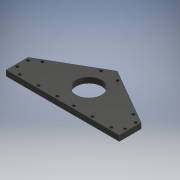
# Autodesk Inventor part: HB04
Saved by Autodesk Inventor 2017 (Build 210142000, 142)
## iProperties
Created: 2019-05-20
Part Number: HB04
Material: Polyethylene, High Density
Document SubType Name: Modeling
Designer: Dell
Density: 0.952 g/cm^3
Appearance: Smooth - Black
Mass: 1258.66 g
Surface Area: 2467.82 cm^2
Volume: 1322.13 cm^3
Author: Dell
Autodesk Inventor part; units mm, degrees
ref_plane "YZ Plane" through (0, 0, 0) normal (1, 0, 0) x (0, 1, 0)
ref_plane "XZ Plane" through (0, 0, 0) normal (0, 1, 0) x (-1, 0, 0)
ref_plane "XY Plane" through (0, 0, 0) normal (0, 0, 1) x (1, 0, 0)
sketch "Sketch1" plane through (0, 0, 0) normal (0, 0, 1) x (1, 0, 0)
  line L0 (262.89, 253.3796) -> (525.78, 101.6)
  line L1 (525.78, 101.6) -> (525.78, -201.9592) construction
  line L2 (525.78, -201.9592) -> (262.89, -353.7388) construction
  line L3 (262.89, -353.7388) -> (0, -201.9592) construction
  line L4 (0, -201.9592) -> (0, 101.6) construction
  line L5 (0, 101.6) -> (262.89, 253.3796)
  line L6 (0, 101.6) -> (0, 0)
  line L7 (0, 0) -> (525.78, 0)
  line L8 (525.78, 0) -> (525.78, 101.6)
  point P0 (262.89, -50.1796)
  dimension "d0" = 525.78
  dimension "d1" = 101.6
  constraints: 18 end point, 2 collinear, 2 point on line, 1 perpendicular, 1 vertical, 13 other
  measures "d0" distance between parallel lines of L4 L1
  measures "d1" distance of L6.end L4.end
extrude "Extrusion1" add sketch "Sketch1" along normal blind 25.4
sketch "Sketch2" plane through (0, 0, 25.4) normal (0, 0, 1) x (1, 0, 0)
  circle A0 centre (262.89, 121.3796) radius 60
  line L0 (0, 0) -> (525.78, 0) projected
  point P0 (262.89, 0)
  dimension "d4" = 121.3796
  dimension "d5" = 120
  constraints: 1 centre point, 1 midpoint, 1 vertical alignment
  measures "d4" distance from line of L0 A0.centre
  measures "d5" diameter of A0
extrude "Extrusion2" cut sketch "Sketch2" against normal through all
sketch "Sketch3" plane through (0, 0, 25.4) normal (0, 0, 1) x (1, 0, 0)
  circle A0 centre (262.89, 121.3796) radius 60 construction
  line L0 (0, 101.6) -> (0, 0) construction
  line L1 (0, 0) -> (525.78, 0) construction
  line L2 (525.78, 0) -> (525.78, 101.6) construction
  line L3 (525.78, 101.6) -> (262.89, 253.3796) construction
  line L4 (262.89, 253.3796) -> (0, 101.6) construction
  line L5 (12.7, 94.2677) -> (12.7, 12.7) construction
  line L6 (12.7, 12.7) -> (513.08, 12.7) construction
  line L7 (513.08, 12.7) -> (513.08, 94.2677) construction
  line L8 (513.08, 94.2677) -> (262.89, 238.7149) construction
  line L9 (262.89, 238.7149) -> (12.7, 94.2677) construction
  circle A1 centre (12.7, 88.5) radius 2
  circle A2 centre (12.7, 38.5) radius 2
  line L10 (12.7, 88.5) -> (12.7, 38.5) construction
  circle A3 centre (51.1925, 116.4913) radius 2
  circle A4 centre (224.3975, 216.4913) radius 2
  circle A5 centre (137.795, 166.4913) radius 2
  circle A6 centre (51.1925, 12.7) radius 2
  circle A7 centre (137.795, 12.7) radius 2
  circle A8 centre (224.3975, 12.7) radius 2
  circle A9 centre (262.89, 12.7) radius 2
  line L11 (51.1925, 116.4913) -> (224.3975, 216.4913) construction
  line L12 (262.89, 238.7149) -> (262.89, 253.3796)
  line L13 (525.78, 101.6) -> (525.78, 0) construction
  line L14 (513.08, 94.2677) -> (513.08, 12.7) construction
  circle A10 centre (513.08, 88.5) radius 2
  circle A11 centre (513.08, 38.5) radius 2
  line L15 (513.08, 88.5) -> (513.08, 38.5) construction
  circle A12 centre (474.5875, 116.4913) radius 2
  circle A13 centre (301.3825, 216.4913) radius 2
  circle A14 centre (387.985, 166.4913) radius 2
  circle A15 centre (474.5875, 12.7) radius 2
  circle A16 centre (387.985, 12.7) radius 2
  circle A17 centre (301.3825, 12.7) radius 2
  circle A18 centre (262.89, 12.7) radius 2
  line L16 (474.5875, 116.4913) -> (301.3825, 216.4913) construction
  line L17 (30.0651, 0) -> (30.0651, 25.4)
  line L18 (30.0651, 25.4) -> (30.0651, 101.6)
  point P0 (525.78, 0)
  point P1 (30.0651, 63.5)
  point P2 (12.7, 63.5)
  dimension "d8" = 12.7
  dimension "d9" = 4
  dimension "d10" = 4
  dimension "d11" = 50
  dimension "d12" = 4
  dimension "d13" = 4
  dimension "d14" = 4
  dimension "d15" = 4
  dimension "d16" = 4
  dimension "d17" = 4
  dimension "d18" = 4
  dimension "d19" = 200
  dimension "d38" = 25.4
  constraints: 28 end point, 18 centre point, 10 point on line, 9 symmetric about line, 5 midpoint, 3 vertical alignment, 2 collinear, 2 horizontal alignment, 2 vertical, 1 perpendicular, 13 other
  measures "d8" distance between parallel lines of L4 L9
  measures "d9" diameter of A1
  measures "d10" diameter of A2
  measures "d11" distance of L10.end L10.start
  measures "d12" diameter of A3
  measures "d13" diameter of A4
  measures "d14" diameter of A5
  measures "d15" diameter of A6
  measures "d16" diameter of A7
  measures "d17" diameter of A8
  measures "d18" diameter of A9
  measures "d19" distance of L11.start L11.end
  measures "d38" distance of L17.start L17.end
extrude "Extrusion3" cut sketch "Sketch3" against normal through all contours A1 | A2 | A3 | A4 | A7 | A8 | A10 | A11 | A12 | A13 | A16 | A17
sketch "Sketch5" plane through (0, 0, 0) normal (0, 0, -1) x (-1, 0, 0)
  circle A0 centre (-513.08, 88.5) radius 2 projected
  circle A1 centre (-387.985, 12.7) radius 2 projected
  circle A2 centre (-224.3975, 216.4913) radius 2 projected
  circle A3 centre (-12.7, 38.5) radius 2 projected
  circle A4 centre (-12.7, 88.5) radius 2 projected
  circle A5 centre (-51.1925, 116.4913) radius 2 projected
  circle A6 centre (-137.795, 12.7) radius 2 projected
  circle A7 centre (-301.3825, 216.4913) radius 2 projected
  circle A8 centre (-474.5875, 116.4913) radius 2 projected
  circle A9 centre (-513.08, 38.5) radius 2 projected
  circle A10 centre (-262.89, 121.3796) radius 60 projected
  line L0 (0, 0) -> (0, 101.6) projected
  line L1 (0, 101.6) -> (-262.89, 253.3796) projected
  line L2 (-262.89, 253.3796) -> (-525.78, 101.6) projected
  line L3 (-525.78, 101.6) -> (-525.78, 0) projected
  line L4 (-525.78, 0) -> (0, 0) projected
  line L5 (-25.4, 25.4) -> (-25.4, 86.9353)
  line L6 (-25.4, 86.9353) -> (-262.89, 224.0502)
  line L7 (-262.89, 224.0502) -> (-500.38, 86.9353)
  line L8 (-500.38, 86.9353) -> (-500.38, 25.4)
  line L9 (-500.38, 25.4) -> (-25.4, 25.4)
  circle A11 centre (-262.89, 121.3796) radius 85.4
  dimension "d26" = 25.4
  dimension "d27" = 25.4
  constraints: 10 end point, 1 centre point, 4 other
  measures "d26" distance between parallel lines of L4 L9
  measures "d27" radial gap between concentric circles of A10 A11
extrude "Extrusion5" cut sketch "Sketch5" against normal blind 19.05 contours L9 L8 L7 L6 L5
sketch "Sketch6" plane through (0, 0, 25.4) normal (0, 0, 1) x (1, 0, 0)
  circle A0 centre (513.08, 38.5) radius 2 construction
  circle A1 centre (513.08, 88.5) radius 2 construction
  circle A2 centre (387.985, 12.7) radius 2 construction
  circle A3 centre (224.3975, 216.4913) radius 2 construction
  circle A4 centre (12.7, 38.5) radius 2 construction
  circle A5 centre (12.7, 88.5) radius 2 construction
  circle A6 centre (51.1925, 116.4913) radius 2 construction
  circle A7 centre (137.795, 12.7) radius 2 construction
  circle A8 centre (301.3825, 216.4913) radius 2 construction
  circle A9 centre (474.5875, 116.4913) radius 2 construction
  circle A10 centre (513.08, 38.5) radius 2 construction
  circle A11 centre (262.89, 121.3796) radius 60 construction
  line L0 (0, 101.6) -> (0, 0) construction
  line L1 (0, 0) -> (525.78, 0) construction
  line L2 (525.78, 0) -> (525.78, 101.6) construction
  line L3 (525.78, 101.6) -> (262.89, 253.3796) construction
  line L4 (262.89, 253.3796) -> (0, 101.6) construction
  circle A12 centre (513.08, 38.5) radius 2 projected
  circle A13 centre (513.08, 38.5) radius 6.5
  circle A14 centre (513.08, 88.5) radius 2 projected
  circle A15 centre (513.08, 88.5) radius 6.5
  circle A16 centre (474.5875, 116.4913) radius 2 projected
  circle A17 centre (474.5875, 116.4913) radius 6.5
  circle A18 centre (301.3825, 216.4913) radius 2 projected
  circle A19 centre (301.3825, 216.4913) radius 6.5
  circle A20 centre (387.985, 12.7) radius 2 projected
  circle A21 centre (387.985, 12.7) radius 6.5
  line L5 (262.89, 253.3796) -> (262.89, 364.4597)
  circle A22 centre (12.7, 88.5) radius 2 construction
  circle A23 centre (12.7, 38.5) radius 6.5
  circle A24 centre (12.7, 88.5) radius 6.5
  circle A25 centre (51.1925, 116.4913) radius 6.5
  circle A26 centre (224.3975, 216.4913) radius 6.5
  circle A27 centre (137.795, 12.7) radius 6.5
  circle A28 centre (224.3975, 12.7) radius 2 projected
  circle A29 centre (301.3825, 12.7) radius 2 projected
  circle A30 centre (224.3975, 12.7) radius 6.5
  circle A31 centre (301.3825, 12.7) radius 6.5
  dimension "d30" = 13
  dimension "d31" = 13
  dimension "d32" = 13
  dimension "d33" = 13
  dimension "d34" = 13
  dimension "d39" = 13
  dimension "d40" = 13
  constraints: 13 centre point, 11 symmetric about line, 8 coincident, 2 end point, 1 vertical, 6 other
  measures "d30" diameter of A13
  measures "d31" diameter of A15
  measures "d32" diameter of A17
  measures "d33" diameter of A19
  measures "d34" diameter of A21
  measures "d39" diameter of A30
  measures "d40" diameter of A31
extrude "Extrusion6" cut sketch "Sketch6" against normal blind 12.7 contours A12 | A13 | A14 | A15 | A16 | A17 | A18 | A19 | A20 | A21 | A23 | A24 | A25 | A26 | A27 | A29 | A30 | A31
sketch "Sketch8" plane through (0, 0, 25.4) normal (0, 0, 1) x (1, 0, 0)
  circle A0 centre (50, 12.7) radius 2
  circle A1 centre (475.78, 12.7) radius 2
  line L0 (0, 101.6) -> (0, 0) projected
  line L1 (525.78, 0) -> (525.78, 101.6) projected
  circle A2 centre (387.985, 12.7) radius 2 projected
  dimension "d41" = 4
  dimension "d42" = 4
  dimension "d43" = 50
  dimension "d44" = 50
  constraints: 2 centre point, 2 horizontal alignment
  measures "d41" diameter of A0
  measures "d42" diameter of A1
  measures "d43" distance from line of L0 A0.centre
  measures "d44" distance from line of L1 A1.centre
extrude "Extrusion7" cut sketch "Sketch8" against normal through all
sketch "Sketch9" plane through (0, 0, 25.4) normal (0, 0, 1) x (1, 0, 0)
  circle A0 centre (50, 12.7) radius 2 projected
  circle A1 centre (475.78, 12.7) radius 2 projected
  circle A2 centre (50, 12.7) radius 6.5
  circle A3 centre (475.78, 12.7) radius 2 projected
  circle A4 centre (475.78, 12.7) radius 6.5
  point P0 (0, 0)
  dimension "d47" = 13
  dimension "d48" = 13
  constraints: 2 centre point, 2 coincident
  measures "d47" diameter of A2
  measures "d48" diameter of A4
extrude "Extrusion8" cut sketch "Sketch9" against normal blind 12.7 contours A0 | A1 | A2 | A4
body "Solid1"
